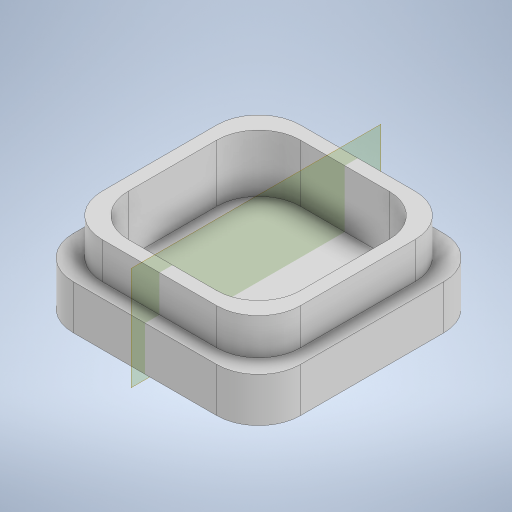
# Autodesk Inventor part: Podstawka_dla_skurwysyna
Saved by Autodesk Inventor 2024 (Build 280153000, 153)
## iProperties
Created: 2023-12-18
Part Number: Podstawka_dla_skurwysyna
Material: Generic
Document SubType Name: Modeling
Designer: Piter
Density: 1 g/cm^3
Appearance: Default
Author: Piter
Autodesk Inventor part; units mm, degrees
ref_plane "YZ Plane" through (0, 0, 0) normal (1, 0, 0) x (0, 1, 0)
ref_plane "XZ Plane" through (0, 0, 0) normal (0, 1, 0) x (-1, 0, 0)
ref_plane "XY Plane" through (0, 0, 0) normal (0, 0, 1) x (1, 0, 0)
sketch "Sketch1" plane through (0, 0, 0) normal (0, 1, 0) x (-1, 0, 0)
  line L0 (-38, 38) -> (38, 38)
  line L1 (38, 38) -> (38, -38)
  line L2 (38, -38) -> (-38, -38)
  line L3 (-38, -38) -> (-38, 38)
  line L4 (-38, 38) -> (38, -38) construction
  line L5 (38, 38) -> (-38, -38) construction
  line L6 (-43.5, 43.5) -> (43.5, 43.5)
  line L7 (43.5, 43.5) -> (43.5, -43.5)
  line L8 (43.5, -43.5) -> (-43.5, -43.5)
  line L9 (-43.5, -43.5) -> (-43.5, 43.5)
  line L10 (-43.5, 43.5) -> (43.5, -43.5) construction
  line L11 (43.5, 43.5) -> (-43.5, -43.5) construction
  point P0 (0, 0)
  dimension "d0" = 76
  dimension "d1" = 76
  dimension "d2" = 87
  dimension "d3" = 87
  constraints: 24 end point, 4 midpoint, 4 parallel, 2 horizontal, 2 perpendicular
  measures "d0" distance of L1.end L2.end
  measures "d1" distance of L0.end L1.end
  measures "d2" distance of L7.end L8.end
  measures "d3" distance of L6.end L7.end
extrude "Extrusion1" add sketch "Sketch1" along normal blind 36 contours L0 L1 L2 L3
extrude "Extrusion2" add sketch "Sketch1" along normal blind 24 contours L0 L1 L2 L3 | L6 L7 L8 L9
sketch "Sketch2" plane through (0, 36, 0) normal (0, 1, 0) x (1, 0, 0)
  line L0 (33, -33) -> (-33, -33)
  line L1 (-33, -33) -> (-33, 33)
  line L2 (-33, 33) -> (33, 33)
  line L3 (33, 33) -> (33, -33)
  line L4 (33, -33) -> (-33, 33) construction
  line L5 (-33, -33) -> (33, 33) construction
  line L6 (-38, 38) -> (-38, -38) projected
  line L7 (38, 38) -> (-38, 38) projected
  point P0 (0, 0)
  dimension "d8" = 5
  dimension "d9" = 5
  constraints: 12 end point, 2 midpoint, 2 parallel, 1 horizontal, 1 perpendicular
  measures "d8" distance between parallel lines of L6 L1
  measures "d9" distance between parallel lines of L7 L2
extrude "Extrusion3" cut sketch "Sketch2" against normal blind 27
fillet "Fillet1" radius 16 12 edges at (38, 30, 38) (38, 30, -38) (-38, 30, -38) (-38, 30, 38) (-43.5, 12, -43.5) (-43.5, 12, 43.5) (43.5, 12, 43.5) (43.5, 12, -43.5) (33, 22.5, 33) (33, 22.5, -33) (-33, 22.5, -33) (-33, 22.5, 33)
ref_plane "Work Plane1" through (0, 0, -27.5) normal (-1, 0, 0) x (0, 0, 1)
move faces "Move1" translate (0, -6, 0) faces at (41.6667, 24, 7.3333)
move faces "Move2" translate (0, -1, 0) faces at (41.6667, 18, -7.3333)
move faces "Move3" translate (0, -5, 0) faces at (5.6667, 36, -36.3333)
body "Solid1"
